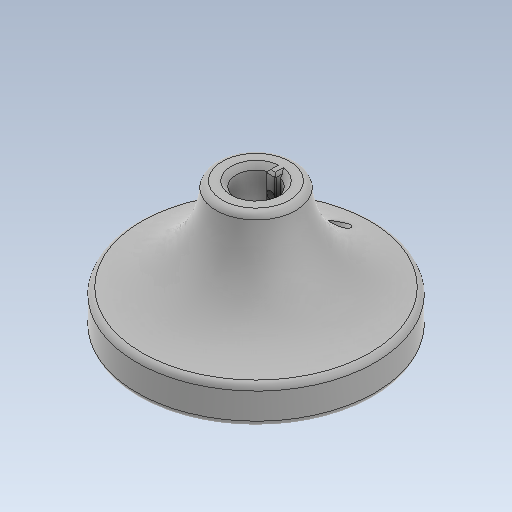
# Autodesk Inventor part: drive_disc
Saved by Autodesk Inventor 2020.2 (Build 242310000, 310)
## iProperties
Created: 2019-10-28
Part Number: drive_disc
Material: PMMA Plastic
Document SubType Name: Modeling
Designer: agmle
Density: 1.188 g/cm^3
Appearance: Smooth - Medium Gray
Mass: 79.3114 g
Surface Area: 167.306 cm^2
Volume: 66.7605 cm^3
Author: agmle
Autodesk Inventor part; units mm, degrees
ref_plane "YZ Plane" through (0, 0, 0) normal (1, 0, 0) x (0, 1, 0)
ref_plane "XZ Plane" through (0, 0, 0) normal (0, 1, 0) x (-1, 0, 0)
sketch "Sketch2" plane through (0, 0, 0) normal (0, 0, 1) x (1, 0, 0)
  line L0 (38.1, 0) -> (38.1, 12)
  line L1 (12.7, 41.75) -> (0, 41.75)
  line L2 (0, 41.75) -> (0, 0) construction
  line L3 (38.1, 0) -> (25.55, 0)
  line L4 (25.55, 0) -> (25.55, 10)
  line L5 (25.55, 10) -> (0, 10)
  line L6 (0, 41.75) -> (0, 10)
  arc A0 (12.7, 41.75) -> (38.1, 12) centre (42.8225, 41.75) ccw
  line L7 (12.7, 41.75) -> (12.7, 12) construction
  line L8 (12.7, 12) -> (38.1, 12) construction
  dimension "d0" = 38.1
  dimension "d1" = 12.7
  dimension "d2" = 12
  dimension "d3" = 12.55
  dimension "d4" = 31.75
  dimension "d5" = 10
  constraints: 18 end point, 3 perpendicular, 2 horizontal, 2 point on circle, 2 point on line, 2 vertical, 1 centre point, 1 collinear, 1 tangent
  measures "d0" distance from line of L2.end L0
  measures "d1" distance of L1.end L1.start
  measures "d2" distance of L0.start L0.end
  measures "d3" distance between parallel lines of L0 L4
  measures "d4" distance of L5.end L1.end
  measures "d5" distance from line of L2.end L5
revolve "Body" add sketch "Sketch2" angle 360 about axis through (0, 41.75, 0) along (0, -1, 0)
sketch "Sketch3" plane through (0, 41.75, 0) normal (0, 1, 0) x (1, 0, 0)
  arc A0 (-1.524, 6.2298) -> (1.524, 6.2298) centre (0, 0) ccw
  line L0 (1.524, 6.2298) -> (1.524, 4.9598)
  line L1 (1.524, 4.9598) -> (1.27, 4.7058)
  line L2 (1.27, 4.7058) -> (-1.27, 4.7058)
  line L3 (-1.27, 4.7058) -> (-1.524, 4.9598)
  line L4 (-1.524, 4.9598) -> (-1.524, 6.2298)
  line L5 (0, 0) -> (0, 4.7058) construction
  dimension "d7" = 12.827
  dimension "d8" = 3.048
  dimension "d9" = 1.524
  dimension "d10" = 0.254
  constraints: 12 end point, 2 equal length, 2 perpendicular, 2 point on circle, 2 vertical, 1 centre point, 1 coincident, 1 midpoint, 1 parallel
  measures "d7" diameter of A0
  measures "d8" distance between parallel lines of L4 L0
  measures "d9" distance from line of L0.start L2
  measures "d10" distance from line of L2 L0.end
extrude "Keyshaft" cut sketch "Sketch3" against normal through all
fillet "Stress Reduction" radius 8 1 edges at (-25.55, 10, 0)
fillet "Softening" radius 2 4 edges at (-25.55, 0, 0) (-38.1, 0, 0) (-38.1, 12, 0) (-12.7, 41.75, 0)
chamfer "Shaft Leadin" distance 1.5875 angle 45 2 edges at (0, 10, 6.4135) (0, 41.75, 6.4135)
chamfer "Key Leadin" distance 0.7937 angle 45 10 edges at (-1.524, 41.75, -6.4072) (-1.397, 41.75, -4.8328) (0, 41.75, -4.7058) (1.397, 41.75, -4.8328) (1.524, 41.75, -6.4072) (1.524, 10, -6.4072) (1.397, 10, -4.8328) (0, 10, -4.7058) (-1.397, 10, -4.8328) (-1.524, 10, -6.4072)
ref_plane "Work Plane1" through (-1.27, 10.7937, -33.2808) normal (0, 0, 1) x (1, 0, 0)
sketch "Sketch5" plane through (-1.27, 10.7937, -33.2808) normal (0, 0, 1) x (1, 0, 0)
  line L0 (1.27, -19.1437) -> (1.27, 39.3062) projected
  line L1 (-9.4923, 30.9563) -> (12.0323, 30.9563) projected
  line L2 (18.82, -0.7937) -> (-16.28, -0.7937) projected
  point P0 (1.27, -10.7937)
  point P1 (1.27, 24.6063)
  point P2 (1.27, 5.5562)
  dimension "d22" = 6.35
  dimension "d23" = 6.35
  constraints: 2 point on line
  measures "d22" distance from line of L1 point (1.27, 24.606)
  measures "d23" distance from line of L2 point (1.27, 5.556)
hole "Grub Screws" at (0, 35.4, -33.2808) at (0, 16.35, -33.2808) direction (0, 0, 1) diameter 2.459 depth 28.575 counterbore diameter 4 counterbore depth 22.225 thread size "M3x0.5" class "6H" standard "ANSI Metric M Profile"
sketch "Sketch6" plane through (0, 0, 0) normal (0, -1, 0) x (1, 0, 0)
  circle A0 centre (0, -31.825) radius 3.1 construction
  line L0 (0, -31.825) -> (0, 0) construction
  line L1 (6.822, -38.1) -> (-7.7809, -38.1) construction
  line L2 (6.2276, -34.925) -> (-8.5536, -34.925) construction
  circle A1 centre (0, 0) radius 38.1 construction
  circle A2 centre (27.5613, -15.9125) radius 3.1 construction
  circle A3 centre (27.5613, 15.9125) radius 3.1 construction
  circle A4 centre (0, 31.825) radius 3.1 construction
  circle A5 centre (-27.5613, 15.9125) radius 3.1 construction
  circle A6 centre (-27.5613, -15.9125) radius 3.1 construction
  dimension "d31" = 6.2
  dimension "d32" = 3.175
  dimension "d35" = 360
  constraints: 6 centre point, 6 coincident, 6 end point, 2 horizontal, 2 tangent, 1 vertical, 19 other
  measures "d31" diameter of A0
  measures "d32" distance between parallel lines of L2 L1
hole "Magnets" at (0, 0, -31.825) at (27.5613, 0, -15.9125) at (27.5613, 0, 15.9125) at (0, 0, 31.825) at (-27.5613, 0, 15.9125) at (-27.5613, 0, -15.9125) direction (0, 1, 0) diameter 6.2 depth 10
chamfer "Leadin" distance 0.5 angle 45 6 edges at (0, 0, -28.725) (-27.5613, 0, -12.8125) (27.5613, 0, -12.8125) (27.5613, 0, 19.0125) (0, 0, 34.925) (-27.5613, 0, 19.0125)
equation "\"d0\" = 0.5 * impeller_od"
equation "\"d1\" = motor_shaft_od"
equation "\"d3\" = magnet_clearance + magnet_od + 2 * magnet_circle_offset"
equation "\"d4\" = motor_shaft_length"
equation "\"d5\" = magnet_length"
equation "\"d8\" = motor_shaft_key"
equation "\"d9\" = 0.5 * motor_shaft_key"
equation "\"d22\" = 0.5 * motor_shaft_od"
equation "\"d23\" = 0.5 * motor_shaft_od"
equation "\"d31\" = magnet_od + magnet_clearance"
equation "\"d32\" = magnet_circle_offset"
equation "\"d37\" = magnet_od + magnet_clearance"
equation "\"d42\" = magnet_length"
equation "\"d44\" = 2 * magnet_clearance"
equation "\"hull_od\" = 219.075"
equation "\"hull_id\" = 201.7268"
equation "\"hull_wall\" = 8.6741"
equation "\"hull_length\" = 609.6"
equation "\"hull_spacing\" = 390.525"
equation "\"impeller_od\" = 76.2"
equation "\"impeller_clearance\" = 0.5"
equation "\"impeller_shaft_id\" = 3.175"
equation "\"impeller_shaft_od\" = 5.715"
equation "\"impeller_shaft_support\" = 3.175"
equation "\"impeller_intake_od\" = 19.05"
equation "\"impeller_vane_thick\" = 2"
equation "\"impeller_vane_inner_rad\" = 3.175"
equation "\"impeller_vane_outer_rad\" = 0.37206"
equation "\"magnet_od\" = 5.95"
equation "\"magnet_length\" = 10"
equation "\"magnet_clearance\" = 0.25"
equation "\"magnet_rad\" = 0.25"
equation "\"magnet_circle_offset\" = 3.175"
equation "\"motor_shaft_od\" = 12.7"
equation "\"motor_shaft_length\" = 31.75"
equation "\"motor_shaft_key\" = 3.048"
equation "\"slab_thick\" = 34.671"
body "Solid1"
